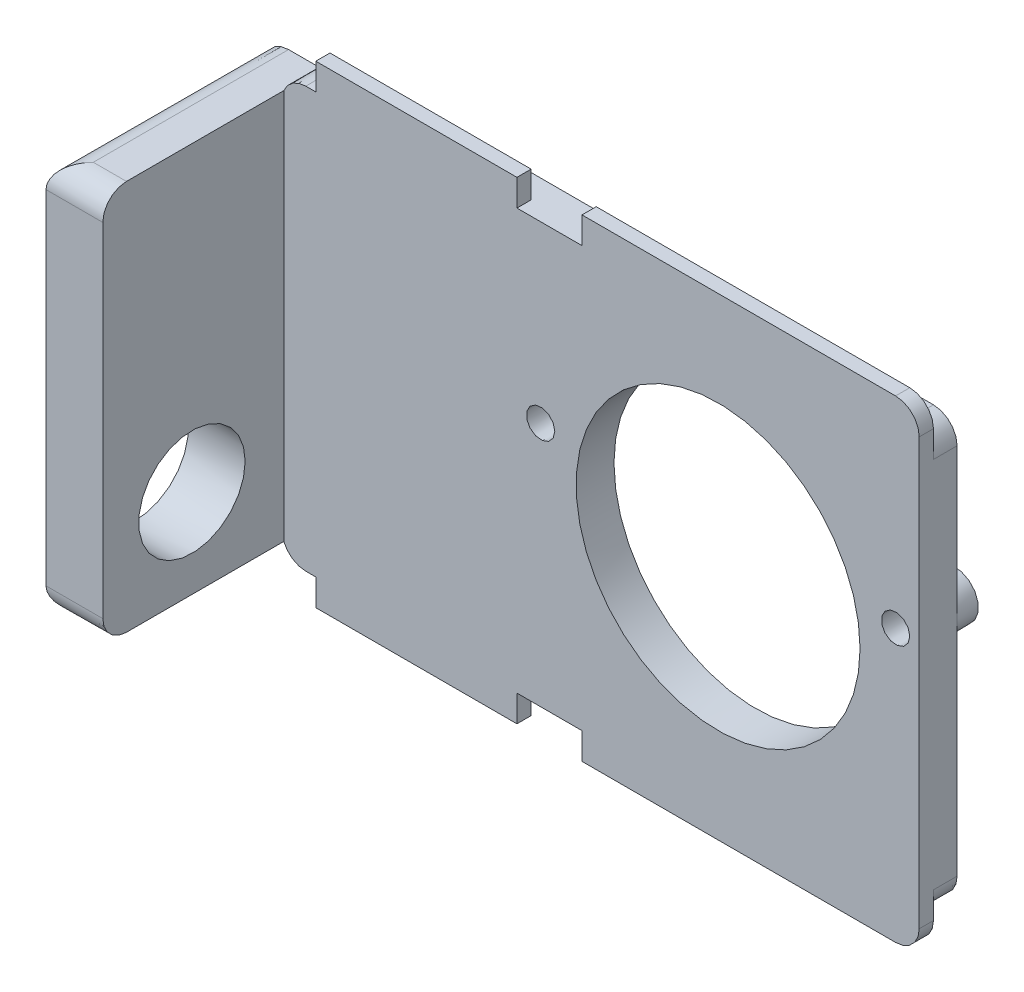
# Autodesk Inventor part: ЛЦМК000002.00.00.00.00.15
Saved by Autodesk Inventor 2021.2 (Build 252289000, 289)
## iProperties
Created: 2025-11-09
Part Number: ЛЦМК000002.00.00.00.00.15
Material: Типовые
Document SubType Name: Modeling
Designer: Захаров
Density: 1 g/cm^3
Appearance: По умолчанию
Author: Захаров
Autodesk Inventor part; units mm, degrees
ref_plane "YZ Plane" through (0, 0, 0) normal (1, 0, 0) x (0, 1, 0)
ref_plane "XZ Plane" through (0, 0, 0) normal (0, 1, 0) x (-1, 0, 0)
ref_plane "XY Plane" through (0, 0, 0) normal (0, 0, 1) x (1, 0, 0)
sketch "Эскиз1" plane through (0, 0, 0) normal (0, 0, 1) x (1, 0, 0)
  line L0 (-26.85, 17.75) -> (26.85, 17.75)
  line L1 (26.85, 17.75) -> (26.85, -17.75)
  line L2 (26.85, -17.75) -> (-26.85, -17.75)
  line L3 (-26.85, -17.75) -> (-26.85, 17.75)
  line L4 (-26.85, 17.75) -> (26.85, -17.75) construction
  line L5 (26.85, 17.75) -> (-26.85, -17.75) construction
  point P0 (0, 0)
  dimension "d0" = 53.7
  dimension "d1" = 35.5
  constraints: 12 end point, 2 midpoint, 2 parallel, 1 horizontal, 1 perpendicular
  measures "d0" distance of L1.end L2.end
  measures "d1" distance of L0.end L1.end
extrude "Выдавливание1" add sketch "Эскиз1" along normal blind 3.2
sketch "Эскиз2" plane through (0, 0, 0) normal (0, 0, -1) x (-1, 0, 0)
  line L0 (31.65, -16.5) -> (26.85, -16.5)
  line L1 (26.85, -16.5) -> (26.85, 16.5)
  line L2 (26.85, 16.5) -> (31.65, 16.5)
  line L3 (31.65, 16.5) -> (31.65, -16.5)
  line L4 (31.65, -16.5) -> (26.85, 16.5) construction
  line L5 (26.85, -16.5) -> (31.65, 16.5) construction
  line L6 (26.85, 17.75) -> (26.85, -17.75) projected
  point P0 (0, 0)
  point P1 (29.25, 0)
  point P2 (26.85, 0)
  dimension "d4" = 4.8
  dimension "d5" = 33
  constraints: 12 end point, 4 midpoint, 2 parallel, 1 horizontal, 1 perpendicular
  measures "d4" distance of L1.end L2.end
  measures "d5" distance of L0.end L1.end
extrude "Выдавливание2" add sketch "Эскиз2" against normal blind 18.5
sketch "Эскиз3" plane through (0, 0, 3.2) normal (0, 0, 1) x (1, 0, 0)
  line L0 (-1.65, 20) -> (26.85, 20)
  line L1 (26.85, 20) -> (26.85, -20)
  line L2 (26.85, -20) -> (-1.65, -20)
  line L3 (-1.65, -20) -> (-1.65, 20)
  line L4 (-1.65, 20) -> (26.85, -20) construction
  line L5 (26.85, 20) -> (-1.65, -20) construction
  line L6 (26.85, -17.75) -> (26.85, 17.75) projected
  line L7 (-24.15, 20) -> (-7.15, 20)
  line L8 (-7.15, 20) -> (-7.15, -20)
  line L9 (-7.15, -20) -> (-24.15, -20)
  line L10 (-24.15, -20) -> (-24.15, 20)
  line L11 (-24.15, 20) -> (-7.15, -20) construction
  line L12 (-7.15, 20) -> (-24.15, -20) construction
  point P0 (0, 0)
  point P1 (12.6, 0)
  point P2 (26.85, 0)
  point P3 (-15.65, 0)
  dimension "d8" = 28.5
  dimension "d9" = 40
  dimension "d10" = 17
  dimension "d11" = 40
  dimension "d12" = 5.5
  constraints: 24 end point, 6 midpoint, 4 parallel, 2 horizontal, 2 perpendicular
  measures "d8" distance of L1.end L2.end
  measures "d9" distance of L0.end L1.end
  measures "d10" distance of L8.end L9.end
  measures "d11" distance of L7.end L8.end
  measures "d12" distance between parallel lines of L8 L3
extrude "Выдавливание3" add sketch "Эскиз3" against normal blind 1.2
sketch "Эскиз4" plane through (0, 0, 0) normal (0, 0, -1) x (-1, 0, 0)
  circle A0 centre (-9.85, 0) radius 12
  line L0 (-26.85, -17.75) -> (-26.85, 17.75) projected
  circle A1 centre (-24.85, 3) radius 2
  circle A2 centre (-24.85, 3) radius 1.2
  line L1 (-9.85, 0) -> (-9.85, 16.0932) construction
  circle A3 centre (5.15, 3) radius 2
  circle A4 centre (5.15, 3) radius 1.2
  line L2 (1.65, 20) -> (-26.85, 20) projected
  point P0 (0, 0)
  dimension "d15" = 24
  dimension "d16" = 17
  dimension "d17" = 4
  dimension "d18" = 2.4
  dimension "d19" = 30
  dimension "d20" = 17
  constraints: 5 centre point, 2 coincident, 2 end point, 2 symmetric about line, 1 horizontal alignment, 1 vertical, 2 other
  measures "d15" diameter of A0
  measures "d16" distance from line of L0 L1.start
  measures "d17" diameter of A1
  measures "d18" diameter of A2
  measures "d19" distance of A3.centre A1.centre
  measures "d20" distance from line of L2 A1.centre
extrude "Выдавливание4" cut sketch "Эскиз4" against normal up to next contours A0
extrude "Выдавливание5" add sketch "Эскиз4" along normal blind 1.8 contours A1 | A3
extrude "Выдавливание6" cut sketch "Эскиз4" against normal up to next contours A2 | A4
sketch "Эскиз5" plane through (-31.65, -16.5, 0) normal (-1, 0, 0) x (0, 0, 1)
  circle A0 centre (10.968, 7.5) radius 4.5
  line L0 (0, 0) -> (18.5, 0) projected
  point P0 (0, 16.5)
  dimension "d27" = 9
  dimension "d28" = 7.5
  constraints: 1 centre point
  measures "d27" diameter of A0
  measures "d28" distance from line of L0 A0.centre
extrude "Выдавливание7" cut sketch "Эскиз5" against normal up to next
fillet "Сопряжение1" radius 2 10 edges at (-29.25, -16.5, 18.5) (-29.25, 16.5, 18.5) (-31.65, -16.5, 9.25) (-31.65, 16.5, 9.25) (26.85, 20, 2.6) (26.85, 17.75, 1) (26.85, -17.75, 1) (26.85, -20, 2.6) (-26.85, 17.75, 1.6) (-26.85, -17.75, 1.6)
